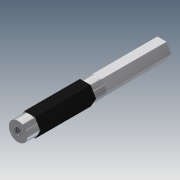
# Autodesk Inventor part: Live Axle
Saved by Autodesk Inventor 2014 SP1 (Build 180222100, 222)
## iProperties
Created: 2013-11-28
Part Number: Live Axle
Material: Aluminum 7075
Document SubType Name: Modeling
Designer: Rauhul Varma
Mass: 31.8188 g
Surface Area: 48.9284 cm^2
Volume: 11.3234 cm^3
Density: 2.81 g/cm^3
Appearance: Aluminum - Polished
Author: Rauhul Varma
Autodesk Inventor part; units mm, degrees
ref_plane "YZ Plane" through (0, 0, 0) normal (1, 0, 0) x (0, 1, 0)
ref_plane "XZ Plane" through (0, 0, 0) normal (0, 1, 0) x (-1, 0, 0)
ref_plane "XY Plane" through (0, 0, 0) normal (0, 0, 1) x (1, 0, 0)
sketch "Sketch1" plane through (0, 0, 0) normal (0, 0, 1) x (1, 0, 0)
  circle A0 centre (0, 0) radius 6.35
  dimension "d0" = 12.7
  constraints: 1 centre point, 1 coincident
  measures "d0" diameter of A0
extrude "Internal 1/2\" Round" add sketch "Sketch1" against normal blind 7.9375
sketch "Sketch2" plane through (0, 0, -7.9375) normal (0, 0, -1) x (-1, 0, 0)
  circle A0 centre (0, 0) radius 6.35 projected
  line L0 (3.6662, 6.35) -> (7.3323, 0)
  line L1 (7.3323, 0) -> (3.6662, -6.35)
  line L2 (3.6662, -6.35) -> (-3.6662, -6.35)
  line L3 (-3.6662, -6.35) -> (-7.3323, 0)
  line L4 (-7.3323, 0) -> (-3.6662, 6.35)
  line L5 (-3.6662, 6.35) -> (3.6662, 6.35)
  constraints: 12 end point, 1 coincident, 1 horizontal, 1 tangent, 13 other
extrude "Pulley 1/2\" Hex" add sketch "Sketch2" along normal blind 38.1
sketch "Sketch3" plane through (0, 0, -46.0375) normal (0, 0, -1) x (-1, 0, 0)
  circle A0 centre (0, 0) radius 6.35
  constraints: 1 centre point, 1 coincident
extrude "External 1/2\" Round" add sketch "Sketch3" along normal blind 7.9375
sketch "Sketch4" plane through (0, 0, -53.975) normal (0, 0, -1) x (-1, 0, 0)
  circle A0 centre (0, 0) radius 6.35 projected
  line L0 (3.2748, 5.4404) -> (6.3489, 0.1158)
  line L1 (6.3489, -0.1158) -> (3.2748, -5.4404)
  line L2 (3.0742, -5.5563) -> (-3.0742, -5.5563)
  line L3 (-3.2748, -5.4404) -> (-6.3489, -0.1158)
  line L4 (-6.3489, 0.1158) -> (-3.2748, 5.4404)
  line L5 (-3.0742, 5.5562) -> (3.0742, 5.5562)
  dimension "d7" = 11.1125
  constraints: 12 end point, 1 coincident, 1 horizontal, 20 other
  measures "d7" distance between parallel lines of L2 L5
extrude "Wheel 7/16\" Hex" add sketch "Sketch4" along normal blind 44.45 contours A0 L1 L2 L3 L4 L5 L0
sketch "Sketch6" plane through (0, 0, -98.425) normal (0, 0, -1) x (-1, 0, 0)
  arc A0 (6.3489, -0.1158) -> (6.3489, 0.1158) centre (0, 0) ccw projected
  constraints: 1 coincident
sketch "Sketch5" plane through (0, 0, 0) normal (0, 0, 1) x (1, 0, 0)
  circle A0 centre (0, 0) radius 6.35 projected
  constraints: 1 coincident
hole "Internal 1/4\"-20 Tap" at (0, 0, 0) direction (0, 0, -1) diameter 4.9784 depth 19.05 tip angle 118 thread size "1/4-20 UNC" class "2B" standard "ANSI Unified Screw Threads"
hole "External 1/4\"-20 Tap" at (0, 0, -98.425) direction (0, 0, 1) diameter 4.9784 depth 19.05 tip angle 118 thread size "1/4-20 UNC" class "2B" standard "ANSI Unified Screw Threads"
body "Solid1"
